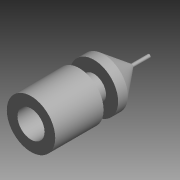
# Autodesk Inventor part: Nozzle
Saved by Autodesk Inventor 2015 (Build 190159000, 159)
## iProperties
Created: 2015-01-06
Part Number: Nozzle
Material: Generic
Document SubType Name: Modeling
Designer: ice
Density: 1 g/cm^3
Appearance: Default
Mass: 1.02114 g
Surface Area: 9.24729 cm^2
Volume: 1.02114 cm^3
Author: ice
Autodesk Inventor part; units mm, degrees
ref_plane "YZ Plane" through (0, 0, 0) normal (1, 0, 0) x (0, 1, 0)
ref_plane "XZ Plane" through (0, 0, 0) normal (0, 1, 0) x (-1, 0, 0)
ref_plane "XY Plane" through (0, 0, 0) normal (0, 0, 1) x (1, 0, 0)
sketch "Sketch1" plane through (0, 0, 0) normal (0, 0, 1) x (1, 0, 0)
  line L0 (-5, -6) -> (-5, 4)
  line L1 (-5, 4) -> (-2.5, 4)
  line L2 (-2.5, 4) -> (-2.5, 7)
  line L3 (-2.5, 7) -> (-5, 7)
  line L4 (-5, 7) -> (-5, 9)
  line L5 (-0.35, 14.8125) -> (-5, 9)
  line L6 (0, 14.375) -> (0, 0)
  line L7 (0, 14.375) -> (0, 18.375)
  line L8 (-0.15, 18.375) -> (-0.35, 18.375)
  line L9 (-0.35, 18.375) -> (-0.35, 14.8125)
  line L10 (-1, 2) -> (-1, 12.1943)
  line L11 (-0.15, 18.375) -> (-0.15, 13.0443)
  arc A0 (-0.15, 13.0443) -> (-1, 12.1943) centre (-0.15, 12.1943) ccw
  line L12 (-2.8, -6) -> (-2.8, 2)
  line L13 (-2.8, 2) -> (-1, 2)
  line L14 (-5, -6) -> (-2.8, -6)
  point P0 (-1, 14)
  point P1 (-0.7, 14.375)
  dimension "d3" = 10
  dimension "d4" = 2.5
  dimension "d5" = 3
  dimension "d7" = 2
  dimension "d55" = 3.5625
  dimension "d58" = 5.8125
  dimension "d59" = 0.35
  dimension "d60" = 0.15
  dimension "d66" = 8
  constraints: 30 end point, 5 point on line, 2 horizontal, 2 point on circle, 1 centre point, 1 perpendicular, 1 vertical
  measures "d3" distance of L0.start L0.end
  measures "d4" distance of L0.end L1.end
  measures "d5" distance of L1.end L2.end
  measures "d7" distance of L3.end L4.end
  measures "d55" distance of L5.start L8.end
  measures "d58" vertical distance of L4.end L5.start
  measures "d59" distance of L7.end L8.end
  measures "d60" distance of L8.start L7.end
  measures "d66" distance of L12.start L12.end
revolve "Revolution1" add sketch "Sketch1" angle 360 about axis through (0, 14.375, 0) along (0, -1, 0)
body "Solid1"
